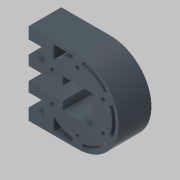
# Autodesk Inventor part: SJ001
Saved by Autodesk Inventor 2017 (Build 210142000, 142)
## iProperties
Created: 2017-06-03
Part Number: SJ001
Material: ABS Plastic
Document SubType Name: Modeling
Designer: Zach
Density: 1.06 g/cm^3
Appearance: CR Dark Blue
Author: Zach
Autodesk Inventor part; units mm, degrees
ref_plane "YZ Plane" through (0, 0, 0) normal (1, 0, 0) x (0, 1, 0)
ref_plane "XZ Plane" through (0, 0, 0) normal (0, 1, 0) x (-1, 0, 0)
ref_plane "XY Plane" through (0, 0, 0) normal (0, 0, 1) x (1, 0, 0)
sketch "Sketch1" plane through (0, 0, 0) normal (0, 0, 1) x (1, 0, 0)
  circle A0 centre (0, 0) radius 62.5 construction
  line L0 (0, 62.5) -> (-75, 62.5)
  line L1 (-75, 62.5) -> (-75, -62.5)
  line L2 (-75, -62.5) -> (0, -62.5)
  arc A1 (0, -62.5) -> (0, 62.5) centre (0, 0) ccw
  dimension "d0" = 125
  dimension "d1" = 75
  dimension "d2" = 75
  constraints: 6 end point, 4 point on circle, 4 tangent, 2 centre point, 1 coincident, 1 concentric, 1 horizontal, 1 perpendicular
  measures "d0" diameter of A0
  measures "d1" distance of L0.start L0.end
  measures "d2" distance of L1.end L2.end
extrude "Extrusion1" add sketch "Sketch1" along normal blind 50
sketch "Sketch6" plane through (0, 0, 50) normal (0, 0, 1) x (1, 0, 0)
  line L0 (-22.5, -22.5) -> (22.5, -22.5)
  line L1 (22.5, -22.5) -> (22.5, 22.5)
  line L2 (22.5, 22.5) -> (-22.5, 22.5)
  line L3 (-22.5, 22.5) -> (-22.5, -22.5)
  line L4 (-22.5, -22.5) -> (22.5, 22.5) construction
  line L5 (22.5, -22.5) -> (-22.5, 22.5) construction
  point P0 (0, 0)
  dimension "d23" = 45
  dimension "d24" = 45
  constraints: 12 end point, 2 midpoint, 2 parallel, 1 horizontal, 1 perpendicular
  measures "d23" distance of L2.end L1.end
  measures "d24" distance of L1.end L0.end
extrude "Extrusion6" cut sketch "Sketch6" against normal blind 40
sketch "Sketch7" plane through (-22.5, -22.5, 50) normal (1, 0, 0) x (0, 0, -1)
  line L0 (40, 32.5) -> (0, 32.5)
  line L1 (0, 32.5) -> (0, 12.5)
  line L2 (0, 12.5) -> (40, 12.5)
  line L3 (40, 12.5) -> (40, 32.5)
  point P0 (50, 22.5)
  point P1 (40, 22.5)
  dimension "d27" = 40
  dimension "d28" = 20
  dimension "d29" = 10
  constraints: 8 end point, 2 parallel, 1 horizontal, 1 horizontal alignment, 1 midpoint, 1 perpendicular
  measures "d27" distance of L2.end L1.end
  measures "d28" distance of L1.end L0.end
  measures "d29" distance from line of point (50, 22.5) L3
extrude "Extrusion7" cut sketch "Sketch7" against normal through all
sketch "Sketch9" plane through (0, 0, 50) normal (0, 0, 1) x (1, 0, 0)
  circle A0 centre (0, 45) radius 2.5
  circle A1 centre (-38.9711, 22.5) radius 2.5
  circle A2 centre (-38.9711, -22.5) radius 2.5
  circle A3 centre (0, -45) radius 2.5
  circle A4 centre (38.9711, -22.5) radius 2.5
  circle A5 centre (38.9711, 22.5) radius 2.5
  point P0 (0, 0)
  dimension "d35" = 5
  dimension "d36" = 45
  dimension "d39" = 360
  constraints: 6 centre point, 13 other
  measures "d35" diameter of A0
  measures "d36" distance of point (0, 0) A0.centre
extrude "Extrusion9" cut sketch "Sketch9" against normal through all
sketch "Sketch10" plane through (0, 0, 50) normal (0, 0, 1) x (1, 0, 0)
  circle A0 centre (0, 0) radius 52.5
  arc A1 (0, -57.5) -> (0, -57.5) centre (0, 0) ccw
  line L0 (0, -57.5) -> (-75, -57.5)
  line L1 (-75, 57.5) -> (-75, -57.5)
  line L2 (0, -57.5) -> (-75, -57.5)
  line L3 (0, 57.5) -> (-75, 57.5)
  circle A2 centre (0, 0) radius 57.5 construction
  arc A3 (0, -57.5) -> (0, 57.5) centre (0, 0) ccw
  line L4 (-75, -10) -> (-75, 10)
  point P0 (-75, 0)
  dimension "d111" = 115
  dimension "d43" = 105
  dimension "d114" = 90
  constraints: 10 end point, 4 point on circle, 3 centre point, 3 coincident, 2 midpoint, 2 tangent, 1 perpendicular, 1 vertical alignment, 2 other
  measures "d43" diameter of A0
  measures "d114" angle of L1 L3
extrude "Extrusion10" cut sketch "Sketch10" against normal blind 40
sketch "Sketch12" plane through (0, 0, 10) normal (0, 0, 1) x (1, 0, 0)
  line L0 (0, 0) -> (77.9423, -45) construction
  line L1 (0, 0) -> (90, 0) construction
  line L2 (48.75, -19.4856) -> (57.4855, -24.529)
  line L3 (41.25, -32.476) -> (49.9855, -37.5194)
  arc A0 (41.25, -32.476) -> (48.75, -19.4856) centre (0, 0) ccw
  arc A1 (49.9877, -37.5164) -> (57.484, -24.5324) centre (-4.3593, 2.5168) ccw
  line L4 (41.25, 32.476) -> (49.9855, 37.5194)
  arc A2 (48.75, 19.4856) -> (41.25, 32.476) centre (0, 0) ccw
  line L5 (48.75, 19.4856) -> (57.4855, 24.529)
  arc A3 (57.4855, 24.529) -> (49.9855, 37.5194) centre (-4.3593, -2.5168) ccw
  line L6 (0, 0) -> (0, -109.4234) construction
  line L7 (7.5, -51.9615) -> (7.5, -62.0484)
  line L8 (-7.5, -51.9615) -> (-7.5, -62.5)
  line L9 (0, -62.5) -> (-7.5, -62.5)
  arc A4 (-7.5, -51.9615) -> (7.5, -51.9615) centre (0, 0) ccw
  line L10 (-7.5, 51.9615) -> (-7.5, 62.5)
  line L11 (0, 62.5) -> (-7.5, 62.5)
  arc A5 (7.5, 51.9615) -> (-7.5, 51.9615) centre (0, 0) ccw
  arc A6 (-51.5388, -10) -> (-51.5388, 10) centre (0, 0) ccw projected
  arc A7 (0, -62.5) -> (0, 62.5) centre (0, 0) ccw projected
  line L12 (-75, -62.5) -> (0, -62.5) construction
  arc A8 (0, -62.5) -> (7.5, -62.0484) centre (0, 0) ccw
  line L13 (7.5, 51.9615) -> (7.5, 62.0484)
  arc A9 (7.5, 62.0484) -> (0, 62.5) centre (0, 0) ccw
  point P0 (54.0974, -31.2332)
  dimension "d50" = 30
  dimension "d52" = 15
  dimension "d53" = 52.5
  dimension "d54" = 67.5
  dimension "d57" = 60
  dimension "d61" = 15
  constraints: 26 end point, 21 point on circle, 8 centre point, 3 concentric, 2 symmetric about line, 2 vertical, 1 equal length, 1 horizontal, 1 parallel, 1 point on line, 14 other
  measures "d50" angle of L0 L1
  measures "d52" distance between parallel lines of L3 L2
  measures "d53" radius of A0
  measures "d54" radius of A1
  measures "d61" distance between parallel lines of L8 L7
extrude "Extrusion11" add sketch "Sketch12" along normal blind 40 contours L2 A7 A1 L3 A0 | A2 L4 A3 L5 | A7 A1 | A3 A7 | L7 A7 L9 L8 A4 | A5 L10 L11 A7 L13
sketch "Sketch16" plane through (0, 0, 10) normal (0, 0, 1) x (1, 0, 0)
  line L0 (-22.5, 10) -> (-51.5388, 10) projected
  line L1 (-51.5388, 10) -> (-51.5388, 62.5)
  line L2 (-36.5388, 62.5) -> (-36.5388, 37.6983)
  arc A0 (-36.5388, 37.6983) -> (-51.5388, 10) centre (0, 0) ccw
  arc A1 (-7.5, 51.9615) -> (-51.5388, 10) centre (0, 0) ccw projected
  line L3 (-36.5388, 62.5) -> (-51.5388, 62.5)
  line L4 (0, 0) -> (-111.9606, 0) construction
  line L5 (-51.5388, -10) -> (-51.5388, -62.5)
  line L6 (-36.5388, -62.5) -> (-36.5388, -37.6983)
  arc A2 (-51.5388, -10) -> (-36.5388, -37.6983) centre (0, 0) ccw
  line L7 (-36.5388, -62.5) -> (-51.5388, -62.5)
  point P0 (-44.0388, -62.5)
  dimension "d69" = 15
  constraints: 14 end point, 4 point on circle, 4 symmetric about line, 2 centre point, 2 vertical, 1 concentric, 1 horizontal, 1 midpoint, 1 other
  measures "d69" distance between parallel lines of L1 L2
extrude "Extrusion14" add sketch "Sketch16" along normal blind 40
sketch "Sketch17" plane through (0, 0, 10) normal (0, 0, 1) x (1, 0, 0)
  line L0 (-51.5388, 57.5) -> (-51.5388, 10) projected
  line L1 (-51.5388, 10) -> (-75, 10)
  line L2 (-75, -57.5) -> (-75, 57.5) projected
  line L3 (-51.5388, 25) -> (-75, 25)
  line L4 (-51.5388, -10) -> (-51.5388, -57.5) projected
  line L5 (-51.5388, -10) -> (-75, -10)
  line L6 (-51.5388, -25) -> (-75, -25)
  line L7 (-51.5388, 25) -> (-51.5388, 10)
  line L8 (-75, 25) -> (-75, 10)
  line L9 (-75, -10) -> (-75, -25)
  line L10 (-51.5388, -10) -> (-51.5388, -25)
  point P0 (0, 0)
  point P1 (-51.5388, 67.5)
  point P2 (-75, -67.5)
  point P3 (-75, 67.5)
  point P4 (-51.5388, -67.5)
  point P5 (-75, -62.5)
  point P6 (-75, 62.5)
  point P7 (-51.5388, 62.5)
  point P8 (-51.5388, -62.5)
  dimension "d72" = 15
  dimension "d73" = 15
  constraints: 16 end point, 4 horizontal, 2 collinear, 2 vertical, 1 point on line, 4 other
  measures "d72" distance between parallel lines of L1 L3
  measures "d73" distance between parallel lines of L6 L5
extrude "Extrusion15" add sketch "Sketch17" along normal blind 40
sketch "Sketch19" plane through (0, 0, 10) normal (0, 0, 1) x (1, 0, 0)
  line L0 (-75, 62.5) -> (-51.5388, 62.5)
  line L1 (-75, 25) -> (-75, -25) projected
  line L2 (-51.5388, 62.5) -> (-75, 62.5)
  line L3 (-75, 62.5) -> (-75, 45)
  line L4 (-75, 45) -> (-51.5388, 45)
  line L5 (-51.5388, 45) -> (-51.5388, 62.5)
  line L6 (-51.5388, -62.5) -> (-75, -62.5)
  line L7 (-75, 62.5) -> (-75, -62.5) projected
  line L8 (-51.5388, -62.5) -> (-75, -62.5)
  line L9 (-75, -62.5) -> (-75, -45)
  line L10 (-75, -45) -> (-51.5388, -45)
  line L11 (-51.5388, -45) -> (-51.5388, -62.5)
  point P0 (0, 0)
  dimension "d84" = 17.5
  dimension "d85" = 17.5
  constraints: 20 end point, 4 parallel, 2 horizontal, 2 perpendicular, 2 point on line
  measures "d84" distance of L3.end L2.end
  measures "d85" distance of L8.end L9.end
extrude "Extrusion16" add sketch "Sketch19" along normal blind 40
sketch "Sketch18" plane through (-75, -62.5, 0) normal (-1, 0, 0) x (0, 0, 1)
  circle A0 centre (40, 45) radius 2.5
  circle A1 centre (20, 45) radius 2.5
  line L0 (50, 52.5) -> (50, 37.5) projected
  line L1 (0, 125) -> (0, 0) projected
  circle A2 centre (40, 80) radius 2.5
  circle A3 centre (20, 80) radius 2.5
  circle A4 centre (20, 116.25) radius 2.5
  circle A5 centre (20, 8.75) radius 2.5
  circle A6 centre (40, 8.75) radius 2.5
  circle A7 centre (40, 116.25) radius 2.5
  line L2 (0, 125) -> (50, 125) projected
  line L3 (10, 87.5) -> (50, 87.5) projected
  line L4 (10, 52.5) -> (50, 52.5) projected
  line L5 (0, 0) -> (50, 0) projected
  point P0 (0, 62.5)
  dimension "d76" = 5
  dimension "d77" = 5
  dimension "d78" = 10
  dimension "d80" = 20
  dimension "d91" = 5
  dimension "d92" = 5
  dimension "d94" = 5
  dimension "d95" = 5
  dimension "d96" = 5
  dimension "d97" = 5
  dimension "d115" = 8.75
  dimension "d116" = 7.5
  dimension "d117" = 7.5
  dimension "d118" = 8.75
  constraints: 8 centre point, 6 vertical alignment, 4 horizontal alignment
  measures "d76" diameter of A0
  measures "d77" diameter of A1
  measures "d78" distance from line of L0 A0.centre
  measures "d80" distance of A1.centre A0.centre
  measures "d91" diameter of A2
  measures "d92" diameter of A3
  measures "d94" diameter of A4
  measures "d95" diameter of A5
  measures "d96" diameter of A6
  measures "d97" diameter of A7
  measures "d115" distance from line of L2 A7.centre
  measures "d116" distance from line of L3 A2.centre
  measures "d117" distance from line of L4 A0.centre
  measures "d118" distance from line of L5 A6.centre
extrude "Extrusion18" cut sketch "Sketch18" against normal blind 25
body "Solid1"
